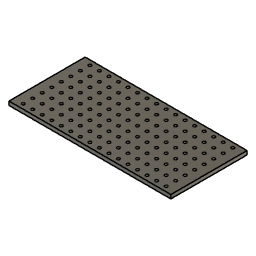
fixated pin holes (Autodesk Fusion 360 design; units mm, degrees)
Autodesk Fusion 360 part; units mm, degrees
sketch "Sketch1" plane through (0, 0, 0) normal (0, 0, 1) x (1, 0, 0)
  line L0 (170, -80) -> (170, 80)
  line L1 (-170, 80) -> (-170, -80)
  line L2 (170, 80) -> (-170, 80)
  line L3 (-170, -80) -> (170, -80)
  ellipse E0 centre (-150, 70.041) end of major axis (-150, 73.041) minor radius 3
  ellipse E1 centre (-150, 50.041) end of major axis (-150, 53.041) minor radius 3
  ellipse E2 centre (-150, 30.041) end of major axis (-150, 33.041) minor radius 3
  ellipse E3 centre (-150, 10.041) end of major axis (-150, 13.041) minor radius 3
  ellipse E4 centre (-150, -9.959) end of major axis (-150, -6.959) minor radius 3
  ellipse E5 centre (-150, -29.959) end of major axis (-150, -26.959) minor radius 3
  ellipse E6 centre (-150, -69.959) end of major axis (-150, -66.959) minor radius 3
  ellipse E7 centre (-150, -49.959) end of major axis (-150, -46.959) minor radius 3
  ellipse E8 centre (-130, 70.041) end of major axis (-130, 73.041) minor radius 3
  ellipse E9 centre (-130, 50.041) end of major axis (-130, 53.041) minor radius 3
  ellipse E10 centre (-130, 30.041) end of major axis (-130, 33.041) minor radius 3
  ellipse E11 centre (-130, 10.041) end of major axis (-130, 13.041) minor radius 3
  ellipse E12 centre (-130, -9.959) end of major axis (-130, -6.959) minor radius 3
  ellipse E13 centre (-130, -29.959) end of major axis (-130, -26.959) minor radius 3
  ellipse E14 centre (-130, -69.959) end of major axis (-130, -66.959) minor radius 3
  ellipse E15 centre (-130, -49.959) end of major axis (-130, -46.959) minor radius 3
  ellipse E16 centre (-110, 70.041) end of major axis (-110, 73.041) minor radius 3
  ellipse E17 centre (-110, 50.041) end of major axis (-110, 53.041) minor radius 3
  ellipse E18 centre (-110, 30.041) end of major axis (-110, 33.041) minor radius 3
  ellipse E19 centre (-110, 10.041) end of major axis (-110, 13.041) minor radius 3
  ellipse E20 centre (-110, -9.959) end of major axis (-110, -6.959) minor radius 3
  ellipse E21 centre (-110, -29.959) end of major axis (-110, -26.959) minor radius 3
  ellipse E22 centre (-110, -69.959) end of major axis (-110, -66.959) minor radius 3
  ellipse E23 centre (-110, -49.959) end of major axis (-110, -46.959) minor radius 3
  ellipse E24 centre (-90, 70.041) end of major axis (-90, 73.041) minor radius 3
  ellipse E25 centre (-90, 50.041) end of major axis (-90, 53.041) minor radius 3
  ellipse E26 centre (-90, 30.041) end of major axis (-90, 33.041) minor radius 3
  ellipse E27 centre (-90, 10.041) end of major axis (-90, 13.041) minor radius 3
  ellipse E28 centre (-90, -9.959) end of major axis (-90, -6.959) minor radius 3
  ellipse E29 centre (-90, -29.959) end of major axis (-90, -26.959) minor radius 3
  ellipse E30 centre (-90, -69.959) end of major axis (-90, -66.959) minor radius 3
  ellipse E31 centre (-90, -49.959) end of major axis (-90, -46.959) minor radius 3
  ellipse E32 centre (-70, 70.041) end of major axis (-70, 73.041) minor radius 3
  ellipse E33 centre (-70, 50.041) end of major axis (-70, 53.041) minor radius 3
  ellipse E34 centre (-70, 30.041) end of major axis (-70, 33.041) minor radius 3
  ellipse E35 centre (-70, 10.041) end of major axis (-70, 13.041) minor radius 3
  ellipse E36 centre (-70, -9.959) end of major axis (-70, -6.959) minor radius 3
  ellipse E37 centre (-70, -29.959) end of major axis (-70, -26.959) minor radius 3
  ellipse E38 centre (-70, -69.959) end of major axis (-70, -66.959) minor radius 3
  ellipse E39 centre (-70, -49.959) end of major axis (-70, -46.959) minor radius 3
  ellipse E40 centre (-50, 70.041) end of major axis (-50, 73.041) minor radius 3
  ellipse E41 centre (-50, 50.041) end of major axis (-50, 53.041) minor radius 3
  ellipse E42 centre (-50, 30.041) end of major axis (-50, 33.041) minor radius 3
  ellipse E43 centre (-50, 10.041) end of major axis (-50, 13.041) minor radius 3
  ellipse E44 centre (-50, -9.959) end of major axis (-50, -6.959) minor radius 3
  ellipse E45 centre (-50, -29.959) end of major axis (-50, -26.959) minor radius 3
  ellipse E46 centre (-50, -69.959) end of major axis (-50, -66.959) minor radius 3
  ellipse E47 centre (-50, -49.959) end of major axis (-50, -46.959) minor radius 3
  ellipse E48 centre (-30, 70.041) end of major axis (-30, 73.041) minor radius 3
  ellipse E49 centre (-30, 50.041) end of major axis (-30, 53.041) minor radius 3
  ellipse E50 centre (-30, 30.041) end of major axis (-30, 33.041) minor radius 3
  ellipse E51 centre (-30, 10.041) end of major axis (-30, 13.041) minor radius 3
  ellipse E52 centre (-30, -9.959) end of major axis (-30, -6.959) minor radius 3
  ellipse E53 centre (-30, -29.959) end of major axis (-30, -26.959) minor radius 3
  ellipse E54 centre (-30, -69.959) end of major axis (-30, -66.959) minor radius 3
  ellipse E55 centre (-30, -49.959) end of major axis (-30, -46.959) minor radius 3
  ellipse E56 centre (-10, 70.041) end of major axis (-10, 73.041) minor radius 3
  ellipse E57 centre (-10, 50.041) end of major axis (-10, 53.041) minor radius 3
  ellipse E58 centre (-10, 30.041) end of major axis (-10, 33.041) minor radius 3
  ellipse E59 centre (-10, 10.041) end of major axis (-10, 13.041) minor radius 3
  ellipse E60 centre (-10, -9.959) end of major axis (-10, -6.959) minor radius 3
  ellipse E61 centre (-10, -29.959) end of major axis (-10, -26.959) minor radius 3
  ellipse E62 centre (-10, -69.959) end of major axis (-10, -66.959) minor radius 3
  ellipse E63 centre (-10, -49.959) end of major axis (-10, -46.959) minor radius 3
  ellipse E64 centre (10, 70.041) end of major axis (10, 73.041) minor radius 3
  ellipse E65 centre (10, 50.041) end of major axis (10, 53.041) minor radius 3
  ellipse E66 centre (10, 30.041) end of major axis (10, 33.041) minor radius 3
  ellipse E67 centre (10, 10.041) end of major axis (10, 13.041) minor radius 3
  ellipse E68 centre (10, -9.959) end of major axis (10, -6.959) minor radius 3
  ellipse E69 centre (10, -29.959) end of major axis (10, -26.959) minor radius 3
  ellipse E70 centre (10, -69.959) end of major axis (10, -66.959) minor radius 3
  ellipse E71 centre (10, -49.959) end of major axis (10, -46.959) minor radius 3
  ellipse E72 centre (30, 70.041) end of major axis (30, 73.041) minor radius 3
  ellipse E73 centre (30, 50.041) end of major axis (30, 53.041) minor radius 3
  ellipse E74 centre (30, 30.041) end of major axis (30, 33.041) minor radius 3
  ellipse E75 centre (30, 10.041) end of major axis (30, 13.041) minor radius 3
  ellipse E76 centre (30, -9.959) end of major axis (30, -6.959) minor radius 3
  ellipse E77 centre (30, -29.959) end of major axis (30, -26.959) minor radius 3
  ellipse E78 centre (30, -69.959) end of major axis (30, -66.959) minor radius 3
  ellipse E79 centre (30, -49.959) end of major axis (30, -46.959) minor radius 3
  ellipse E80 centre (50, 70.041) end of major axis (50, 73.041) minor radius 3
  ellipse E81 centre (50, 50.041) end of major axis (50, 53.041) minor radius 3
  ellipse E82 centre (50, 30.041) end of major axis (50, 33.041) minor radius 3
  ellipse E83 centre (50, 10.041) end of major axis (50, 13.041) minor radius 3
  ellipse E84 centre (50, -9.959) end of major axis (50, -6.959) minor radius 3
  ellipse E85 centre (50, -29.959) end of major axis (50, -26.959) minor radius 3
  ellipse E86 centre (50, -69.959) end of major axis (50, -66.959) minor radius 3
  ellipse E87 centre (50, -49.959) end of major axis (50, -46.959) minor radius 3
  ellipse E88 centre (70, 70.041) end of major axis (70, 73.041) minor radius 3
  ellipse E89 centre (70, 50.041) end of major axis (70, 53.041) minor radius 3
  ellipse E90 centre (70, 30.041) end of major axis (70, 33.041) minor radius 3
  ellipse E91 centre (70, 10.041) end of major axis (70, 13.041) minor radius 3
  ellipse E92 centre (70, -9.959) end of major axis (70, -6.959) minor radius 3
  ellipse E93 centre (70, -29.959) end of major axis (70, -26.959) minor radius 3
  ellipse E94 centre (70, -69.959) end of major axis (70, -66.959) minor radius 3
  ellipse E95 centre (70, -49.959) end of major axis (70, -46.959) minor radius 3
  ellipse E96 centre (90, 70.041) end of major axis (90, 73.041) minor radius 3
  ellipse E97 centre (90, 50.041) end of major axis (90, 53.041) minor radius 3
  ellipse E98 centre (90, 30.041) end of major axis (90, 33.041) minor radius 3
  ellipse E99 centre (90, 10.041) end of major axis (90, 13.041) minor radius 3
  ellipse E100 centre (90, -9.959) end of major axis (90, -6.959) minor radius 3
  ellipse E101 centre (90, -29.959) end of major axis (90, -26.959) minor radius 3
  ellipse E102 centre (90, -69.959) end of major axis (90, -66.959) minor radius 3
  ellipse E103 centre (90, -49.959) end of major axis (90, -46.959) minor radius 3
  ellipse E104 centre (110, 70.041) end of major axis (110, 73.041) minor radius 3
  ellipse E105 centre (110, 50.041) end of major axis (110, 53.041) minor radius 3
  ellipse E106 centre (110, 30.041) end of major axis (110, 33.041) minor radius 3
  ellipse E107 centre (110, 10.041) end of major axis (110, 13.041) minor radius 3
  ellipse E108 centre (110, -9.959) end of major axis (110, -6.959) minor radius 3
  ellipse E109 centre (110, -29.959) end of major axis (110, -26.959) minor radius 3
  ellipse E110 centre (110, -69.959) end of major axis (110, -66.959) minor radius 3
  ellipse E111 centre (110, -49.959) end of major axis (110, -46.959) minor radius 3
  ellipse E112 centre (130, 70.041) end of major axis (130, 73.041) minor radius 3
  ellipse E113 centre (130, 50.041) end of major axis (130, 53.041) minor radius 3
  ellipse E114 centre (130, 30.041) end of major axis (130, 33.041) minor radius 3
  ellipse E115 centre (130, 10.041) end of major axis (130, 13.041) minor radius 3
  ellipse E116 centre (130, -9.959) end of major axis (130, -6.959) minor radius 3
  ellipse E117 centre (130, -29.959) end of major axis (130, -26.959) minor radius 3
  ellipse E118 centre (130, -69.959) end of major axis (130, -66.959) minor radius 3
  ellipse E119 centre (130, -49.959) end of major axis (130, -46.959) minor radius 3
  ellipse E120 centre (150, 70.041) end of major axis (150, 73.041) minor radius 3
  ellipse E121 centre (150, 50.041) end of major axis (150, 53.041) minor radius 3
  ellipse E122 centre (150, 30.041) end of major axis (150, 33.041) minor radius 3
  ellipse E123 centre (150, 10.041) end of major axis (150, 13.041) minor radius 3
  ellipse E124 centre (150, -9.959) end of major axis (150, -6.959) minor radius 3
  ellipse E125 centre (150, -29.959) end of major axis (150, -26.959) minor radius 3
  ellipse E126 centre (150, -69.959) end of major axis (150, -66.959) minor radius 3
  ellipse E127 centre (150, -49.959) end of major axis (150, -46.959) minor radius 3
extrude "Extrude1" add sketch "Sketch1" along normal blind 8
